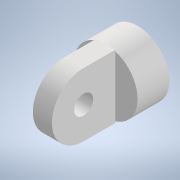
# Autodesk Inventor part: pm connector
Saved by Autodesk Inventor 2021 (Build 250183000, 183)
## iProperties
Created: 2021-05-05
Part Number: pm connector
Material: Generic
Document SubType Name: Modeling
Designer: techv
Density: 1 g/cm^3
Appearance: Default
Author: techv
Autodesk Inventor part; units mm, degrees
ref_plane "YZ Plane" through (0, 0, 0) normal (1, 0, 0) x (0, 1, 0)
ref_plane "XZ Plane" through (0, 0, 0) normal (0, 1, 0) x (-1, 0, 0)
ref_plane "XY Plane" through (0, 0, 0) normal (0, 0, 1) x (1, 0, 0)
sketch "Sketch1" plane through (0, 0, 0) normal (0, 0, 1) x (1, 0, 0)
  circle A0 centre (0, 0) radius 5
  dimension "d0" = 10
  constraints: 1 centre point, 1 coincident
  measures "d0" diameter of A0
extrude "Extrusion1" add sketch "Sketch1" along normal blind 5
sketch "Sketch2" plane through (0, 0, 5) normal (0, 0, 1) x (1, 0, 0)
  line L0 (-1.5, -5) -> (1.5, -5)
  line L1 (1.5, -5) -> (1.5, 5)
  line L2 (1.5, 5) -> (-1.5, 5)
  line L3 (-1.5, 5) -> (-1.5, -5)
  line L4 (-1.5, -5) -> (1.5, 5) construction
  line L5 (1.5, -5) -> (-1.5, 5) construction
  circle A0 centre (0, 0) radius 5 projected
  dimension "d3" = 3
  dimension "d4" = 10
  constraints: 12 end point, 2 midpoint, 2 parallel, 1 horizontal, 1 perpendicular
  measures "d3" distance of L2.end L1.end
  measures "d4" distance of L1.end L0.end
extrude "Extrusion2" add sketch "Sketch2" along normal blind 10 contours L3 A0 L0 | A0 L1 L0 | A0 L3 L1 | L3 L2 A0 | A0 L2 L1
sketch "Sketch3" plane through (1.5, -4.7697, 5) normal (1, 0, 0) x (0, 0, -1)
  line L0 (0, -0.2303) -> (-10, -0.2303) projected
  line L1 (-10, 9.7697) -> (0, -0.2303)
  line L2 (0, -0.2303) -> (0, 9.7697)
  line L3 (-10, 9.7697) -> (-10, -0.2303) projected
  line L4 (0, 9.7697) -> (-10, -0.2303)
  circle A0 centre (-5, 4.7697) radius 1.5
  point P0 (5, 4.7697)
  dimension "d7" = 3
  constraints: 6 end point, 2 perpendicular, 1 centre point, 1 midpoint
  measures "d7" diameter of A0
extrude "Extrusion3" cut sketch "Sketch3" against normal through all contours A0 L4 L1 | L1 L4 A0 | A0 L1 L4 | L1 A0 L4
sketch "Sketch4" plane through (1.5, -4.7697, 5) normal (1, 0, 0) x (0, 0, -1)
  circle A0 centre (-5, 4.7697) radius 1.5 projected
  circle A1 centre (-5, 4.7697) radius 5
  line L0 (-5, 4.7697) -> (-5, 9.7697)
  line L1 (-5, 4.7697) -> (-5, -0.2303)
  line L2 (0, -0.2303) -> (-10, -0.2303) projected
  line L3 (-10, -0.2303) -> (-10, 9.7697) projected
  line L4 (0, 9.7697) -> (-10, 9.7697) projected
  point P0 (5, 4.7697)
  point P1 (-10, 4.7697)
  constraints: 4 end point, 1 coincident, 1 midpoint, 1 vertical, 3 other
extrude "Extrusion4" cut sketch "Sketch4" against normal through all contours A1 L3 L4 | L2 L3 A1
body "Solid1"
